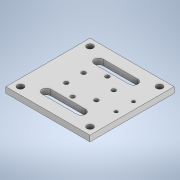
# Autodesk Inventor part: Table
Saved by Autodesk Inventor 2020 (Build 240168000, 168)
## iProperties
Created: 2019-11-16
Part Number: Table
Material: Generic
Document SubType Name: Modeling
Designer: ROBERTO
Density: 1 g/cm^3
Appearance: Default
Author: ROBERTO
Autodesk Inventor part; units mm, degrees
ref_plane "YZ Plane" through (0, 0, 0) normal (1, 0, 0) x (0, 1, 0)
ref_plane "XZ Plane" through (0, 0, 0) normal (0, 1, 0) x (-1, 0, 0)
ref_plane "XY Plane" through (0, 0, 0) normal (0, 0, 1) x (1, 0, 0)
sketch "Sketch1" plane through (0, 0, 0) normal (0, 1, 0) x (-1, 0, 0)
  line L0 (23.0187, -23.0187) -> (-23.0187, -23.0187)
  line L1 (-23.0187, -23.0187) -> (-23.0187, 23.0187)
  line L2 (-23.0187, 23.0187) -> (23.0187, 23.0187)
  line L3 (23.0187, 23.0187) -> (23.0187, -23.0187)
  line L4 (23.0187, -23.0187) -> (-23.0187, 23.0187) construction
  line L5 (-23.0187, -23.0187) -> (23.0187, 23.0187) construction
  line L6 (9.525, -14.2875) -> (-9.525, -14.2875) construction
  line L7 (9.525, -11.9062) -> (-9.525, -11.9062)
  line L8 (-9.525, -16.6688) -> (9.525, -16.6688)
  arc A0 (9.525, -16.6688) -> (9.525, -11.9062) centre (9.525, -14.2875) ccw
  arc A1 (-9.525, -11.9062) -> (-9.525, -16.6688) centre (-9.525, -14.2875) ccw
  line L9 (0, -32.2263) -> (0, 32.2263) construction
  line L10 (32.2263, 0) -> (-32.2263, 0) construction
  line L11 (9.525, 14.2875) -> (-9.525, 14.2875) construction
  line L12 (9.525, 11.9062) -> (-9.525, 11.9062)
  line L13 (-9.525, 16.6688) -> (9.525, 16.6688)
  arc A2 (9.525, 11.9062) -> (9.525, 16.6688) centre (9.525, 14.2875) ccw
  arc A3 (-9.525, 16.6688) -> (-9.525, 11.9062) centre (-9.525, 14.2875) ccw
  point P0 (0, 0)
  point P1 (0, -14.2875)
  point P2 (0, 14.2875)
  dimension "d0" = 46.0375
  dimension "d1" = 46.0375
  dimension "d2" = 19.05
  dimension "d3" = 4.7625
  dimension "d4" = 11.9062
  dimension "d5" = 11.9062
  constraints: 28 end point, 8 point on circle, 7 symmetric about line, 4 centre point, 4 tangent, 3 midpoint, 3 parallel, 2 horizontal, 1 perpendicular, 1 point on line, 2 other
  measures "d0" distance of L1.end L2.end
  measures "d1" distance of L0.end L1.end
  measures "d2" distance of L6.start L6.end
  measures "d3" diameter of A1
  measures "d4" distance between parallel lines of L7 L10
  measures "d5" distance between parallel lines of L12 L10
extrude "Extrusion1" add sketch "Sketch1" along normal blind 3.175
sketch "Sketch2" plane through (0, 3.175, 0) normal (0, 1, 0) x (1, 0, 0)
  line L0 (-23.0187, -23.0187) -> (23.0187, -23.0187) construction
  line L1 (23.0187, -23.0187) -> (23.0187, 23.0187) construction
  line L2 (23.0187, 23.0187) -> (-23.0187, 23.0187) construction
  line L3 (-23.0187, 23.0187) -> (-23.0187, -23.0187) construction
  line L4 (9.525, 11.9062) -> (-9.525, 11.9062) construction
  arc A0 (-9.525, 16.6688) -> (-9.525, 11.9062) centre (-9.525, 14.2875) ccw construction
  line L5 (-9.525, 16.6688) -> (9.525, 16.6688) construction
  arc A1 (9.525, 11.9062) -> (9.525, 16.6688) centre (9.525, 14.2875) ccw construction
  line L6 (9.525, -16.6688) -> (-9.525, -16.6688) construction
  arc A2 (-9.525, -11.9062) -> (-9.525, -16.6688) centre (-9.525, -14.2875) ccw construction
  line L7 (-9.525, -11.9062) -> (9.525, -11.9062) construction
  arc A3 (9.525, -16.6688) -> (9.525, -11.9062) centre (9.525, -14.2875) ccw construction
  circle A4 centre (0, 0) radius 9.525 construction
  line L8 (0, 32.2263) -> (0, -32.2263) construction
  point P0 (0, 9.525)
  dimension "d8" = 19.05
  constraints: 1 coincident, 1 point on line, 1 vertical alignment, 2 other
hole "Hole1" at (0, 3.175, -9.525) direction (0, -1, 0) diameter 2.2606 end through all
pattern_circular "Circular Pattern1" count 6 over 360 about axis through (0, -10, 0) along (0, 1, 0) of "Hole1"
sketch "Sketch4" plane through (0, 3.175, 0) normal (0, 1, 0) x (1, 0, 0)
  circle A0 centre (-19.05, 19.05) radius 1.7272
  circle A1 centre (19.05, 19.05) radius 1.7272
  circle A2 centre (8.2489, 4.7625) radius 1.1303 construction
  circle A3 centre (8.2489, -4.7625) radius 1.1303 construction
  circle A4 centre (0, -9.525) radius 1.1303 construction
  circle A5 centre (-8.2489, -4.7625) radius 1.1303 construction
  circle A6 centre (-8.2489, 4.7625) radius 1.1303 construction
  circle A7 centre (0, 9.525) radius 1.1303 construction
  line L0 (-23.0187, -23.0187) -> (23.0187, -23.0187) construction
  line L1 (23.0187, -23.0187) -> (23.0187, 23.0187) construction
  line L2 (23.0187, 23.0187) -> (-23.0187, 23.0187) construction
  line L3 (-23.0187, 23.0187) -> (-23.0187, -23.0187) construction
  line L4 (9.525, 11.9062) -> (-9.525, 11.9062) construction
  arc A8 (-9.525, 16.6688) -> (-9.525, 11.9062) centre (-9.525, 14.2875) ccw construction
  line L5 (-9.525, 16.6688) -> (9.525, 16.6688) construction
  arc A9 (9.525, 11.9062) -> (9.525, 16.6688) centre (9.525, 14.2875) ccw construction
  line L6 (9.525, -16.6688) -> (-9.525, -16.6688) construction
  arc A10 (-9.525, -11.9062) -> (-9.525, -16.6688) centre (-9.525, -14.2875) ccw construction
  line L7 (-9.525, -11.9062) -> (9.525, -11.9062) construction
  arc A11 (9.525, -16.6688) -> (9.525, -11.9062) centre (9.525, -14.2875) ccw construction
  line L8 (0, 32.2263) -> (0, -32.2263) construction
  line L9 (-32.2263, 0) -> (32.2263, 0) construction
  circle A12 centre (-19.05, -19.05) radius 1.7272
  circle A13 centre (19.05, -19.05) radius 1.7272
  point P0 (0, 0)
  dimension "d19" = 3.4544
  dimension "d20" = 38.1
  dimension "d21" = 19.05
  dimension "d22" = 38.1
  dimension "d23" = 38.1
  constraints: 4 centre point, 2 symmetric about line, 1 equal radius, 2 other
  measures "d19" diameter of A0
  measures "d20" distance of A1.centre A0.centre
  measures "d21" distance from line of A1.centre L8
  measures "d22" distance of A12.centre A0.centre
  measures "d23" distance of A13.centre A1.centre
extrude "Extrusion2" cut sketch "Sketch4" against normal blind 3.175
sketch "Sketch5" plane through (0, 3.175, 0) normal (0, 1, 0) x (1, 0, 0)
  circle A0 centre (-19.05, -19.05) radius 1.7272 construction
  circle A1 centre (19.05, 19.05) radius 1.7272 construction
  circle A2 centre (19.05, -19.05) radius 1.7272 construction
  circle A3 centre (-19.05, 19.05) radius 1.7272 construction
  circle A4 centre (8.2489, 4.7625) radius 1.1303 construction
  circle A5 centre (8.2489, -4.7625) radius 1.1303 construction
  circle A6 centre (0, -9.525) radius 1.1303 construction
  circle A7 centre (-8.2489, -4.7625) radius 1.1303 construction
  circle A8 centre (-8.2489, 4.7625) radius 1.1303 construction
  circle A9 centre (0, 9.525) radius 1.1303 construction
  line L0 (-23.0187, -23.0187) -> (23.0187, -23.0187) construction
  line L1 (23.0187, -23.0187) -> (23.0187, 23.0187) construction
  line L2 (23.0187, 23.0187) -> (-23.0187, 23.0187) construction
  line L3 (-23.0187, 23.0187) -> (-23.0187, -23.0187) construction
  line L4 (9.525, 11.9062) -> (-9.525, 11.9062) construction
  arc A10 (-9.525, 16.6688) -> (-9.525, 11.9062) centre (-9.525, 14.2875) ccw construction
  line L5 (-9.525, 16.6688) -> (9.525, 16.6688) construction
  arc A11 (9.525, 11.9062) -> (9.525, 16.6688) centre (9.525, 14.2875) ccw construction
  line L6 (9.525, -16.6688) -> (-9.525, -16.6688) construction
  arc A12 (-9.525, -11.9062) -> (-9.525, -16.6688) centre (-9.525, -14.2875) ccw construction
  line L7 (-9.525, -11.9062) -> (9.525, -11.9062) construction
  arc A13 (9.525, -16.6688) -> (9.525, -11.9062) centre (9.525, -14.2875) ccw construction
  line L8 (-32.2263, 0) -> (32.2263, 0) construction
  line L9 (0, 32.2263) -> (0, -32.2263) construction
  circle A14 centre (19.05, -19.05) radius 1.7272 construction
  line L10 (19.05, 19.05) -> (19.05, -19.05) construction
  point P0 (0, 0)
  point P1 (19.05, 4.7625)
  point P2 (19.05, -4.7625)
  dimension "d26" = 9.525
  dimension "d27" = 4.7625
  constraints: 2 end point, 1 point on line, 1 vertical
  measures "d26" distance of point (19.05, -4.763) point (19.05, 4.763)
  measures "d27" distance from line of point (19.05, 4.763) L8
hole "Hole2" at (19.05, 3.175, -4.7625) at (19.05, 3.175, 4.7625) direction (0, -1, 0) diameter 1.6942 end through all thread size "2-56 UNC" class "2B" standard "ANSI Unified Screw Threads"
equation "\"d21\" = 0.5 * d20"
equation "\"d27\" = 0.5 * d26"
body "Solid1"
